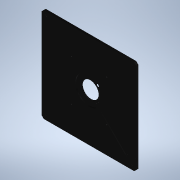
# Autodesk Inventor part: J002949
Saved by Autodesk Inventor 2020.3 (Build 243373000, 373)
## iProperties
RuleStatus: InUse
AfterDocSave0: file://Part Number Cleaner
Created: 2013-12-12
Material: ALUMINUM, 6061-T651
Vendor: HHMI: JFRC - ID&F
Document SubType Name: Modeling
Designer: TABACHNIKT
Density: 2.7 g/cm^3
Mass: 1277.78 g
Surface Area: 1603.58 cm^2
Volume: 473.251 cm^3
Project: P-208804
Description: BASE PLATE
Part Number: J002949
Appearance: Glossy - Black
LAB/DEPT: BRANSON (LAB)
REQUESTING SCIENTIST: ROBIE, ALICE
SURFACE ROUGHNESS: 63 Ra
DESIGN DEPARTMENT: HHMI: JRC - ID&F
SPECIAL FINISH: ANODIZE PER MIL-A-8625F, TYPE II, CLASS 2 (BLACK)
ALTERED ITEM PART NUMBER: N/A
ALTERED ITEM VENDOR: N/A
ALTERED ITEM DESCRIPTION: N/A
PART NUMBER - LEGACY: J002588
Revision Number: A
Autodesk Inventor part; units mm, degrees
ref_plane "YZ Plane" through (0, 0, 0) normal (1, 0, 0) x (0, 1, 0)
ref_plane "XZ Plane" through (0, 0, 0) normal (0, 1, 0) x (-1, 0, 0)
ref_plane "XY Plane" through (0, 0, 0) normal (0, 0, 1) x (1, 0, 0)
sketch "Sketch1" plane through (0, 0, 0) normal (0, 0, 1) x (1, 0, 0)
  line L0 (-152.4, 152.4) -> (152.4, 152.4)
  line L1 (152.4, 152.4) -> (152.4, -152.4)
  line L2 (152.4, -152.4) -> (-152.4, -152.4)
  line L3 (-152.4, -152.4) -> (-152.4, 152.4)
  circle A0 centre (0, 0) radius 26.67
  circle A1 centre (-139.7, 139.7) radius 3.2639
  circle A2 centre (139.7, 139.7) radius 3.2639
  circle A3 centre (139.7, -139.7) radius 3.2639
  circle A4 centre (-139.7, -139.7) radius 3.2639
  point P0 (0, 152.4)
  point P1 (-152.4, 0)
  dimension "d0" = 53.34
  dimension "d1" = 304.8
  dimension "d2" = 304.8
  dimension "d3" = 6.5278
  dimension "d4" = 6.5278
  dimension "d5" = 6.5278
  dimension "d6" = 6.5278
  dimension "d7" = 279.4
  dimension "d8" = 139.7
  dimension "d9" = 279.4
  dimension "d10" = 139.7
  constraints: 8 end point, 5 centre point, 3 horizontal alignment, 3 vertical alignment, 2 midpoint, 2 parallel, 1 coincident, 1 horizontal, 1 perpendicular
  measures "d0" diameter of A0
  measures "d1" distance of L2.end L0.start
  measures "d2" distance of L1.end L2.end
  measures "d3" diameter of A1
  measures "d4" diameter of A2
  measures "d5" diameter of A3
  measures "d6" diameter of A4
  measures "d7" distance of A4.centre A1.centre
  measures "d8" horizontal distance of A4.centre point (0, 0)
  measures "d9" distance of A2.centre A1.centre
  measures "d10" horizontal distance of point (0, 0) A1.centre
extrude "Extrusion1" add sketch "Sketch1" along normal blind 6.35
chamfer "Chamfer1" distance 6.35 angle 45 4 edges at (152.4, 152.4, 3.175) (152.4, -152.4, 3.175) (-152.4, 152.4, 3.175) (-152.4, -152.4, 3.175)
sketch "Sketch10" plane through (0, 0, 6.35) normal (0, 0, 1) x (1, 0, 0)
  line L0 (-213.36, 0) -> (213.36, 0) construction
  line L1 (0, -213.36) -> (0, 213.36) construction
  line L2 (-81.3558, 81.3558) -> (81.3558, -81.3558) construction
  line L3 (15.2664, -26.0427) -> (26.0427, -15.2664) construction
  line L4 (26.0427, -15.2664) -> (33.2269, -22.4506) construction
  line L5 (27.8388, -27.8388) -> (22.4506, -33.2269) construction
  line L6 (22.4506, -33.2269) -> (15.2664, -26.0427) construction
  circle A0 centre (0, 0) radius 26.67 projected
  line L7 (18.8585, -29.6348) -> (29.6348, -18.8585) construction
  line L8 (152.4, 146.05) -> (152.4, -146.05) projected
  line L9 (152.4, -112.6871) -> (120.0658, -112.6871)
  line L10 (116.8908, -115.8621) -> (116.8908, -122.2375)
  line L11 (120.0658, -125.4125) -> (152.4, -125.4125)
  line L12 (152.4, -125.4125) -> (152.4, -112.6871)
  arc A1 (120.0658, -112.6871) -> (116.8908, -115.8621) centre (120.0658, -115.8621) ccw
  arc A2 (116.8908, -122.2375) -> (120.0658, -125.4125) centre (120.0658, -122.2375) ccw
  line L13 (146.05, -152.4) -> (-146.05, -152.4) projected
  line L14 (118.491, -123.8123) -> (150.241, -123.8123) construction
  line L15 (150.241, -123.8123) -> (150.241, -114.2873) construction
  line L16 (150.241, -114.2873) -> (118.491, -114.2873) construction
  line L17 (118.491, -114.2873) -> (118.491, -123.8123) construction
  line L18 (134.366, -114.2873) -> (134.366, -123.8123) construction
  line L19 (118.491, -119.0498) -> (150.241, -119.0498) construction
  arc A3 (33.5957, -29.1055) -> (29.1055, -33.5957) centre (0, 0) ccw
  line L20 (29.1055, -33.5957) -> (116.8908, -121.3809)
  line L21 (33.5957, -29.1055) -> (117.9685, -113.4784)
  line L22 (21.9118, -20.8342) -> (24.0671, -22.9895)
  line L23 (24.0671, -22.9895) -> (22.9895, -24.0671)
  line L24 (22.9895, -24.0671) -> (20.8342, -21.9118)
  line L25 (20.8342, -21.9118) -> (21.9118, -20.8342)
  line L26 (21.373, -21.373) -> (23.5283, -23.5283) construction
  line L27 (20.1158, -22.6302) -> (22.271, -24.7855)
  line L28 (19.0381, -23.7079) -> (20.1158, -22.6302)
  line L29 (21.1934, -25.8631) -> (19.0381, -23.7079)
  line L30 (22.271, -24.7855) -> (21.1934, -25.8631)
  line L31 (22.6302, -20.1158) -> (23.7079, -19.0381)
  line L32 (24.7855, -22.271) -> (22.6302, -20.1158)
  line L33 (23.7079, -19.0381) -> (25.8631, -21.1934)
  line L34 (25.8631, -21.1934) -> (24.7855, -22.271)
  point P0 (22.3249, -22.3249)
  point P1 (20.6546, -27.8388)
  point P2 (27.8388, -20.6546)
  point P3 (121.666, -119.0498)
  point P4 (147.066, -119.0498)
  point P5 (20.5289, -24.121)
  point P6 (24.121, -20.5289)
  point P7 (19.577, -23.1691)
  point P8 (21.7322, -25.3243)
  point P9 (23.1691, -19.577)
  point P10 (25.3243, -21.7322)
  dimension "d84" = 45
  dimension "d85" = 10.16
  dimension "d86" = 15.24
  dimension "d87" = 39.37
  dimension "d90" = 2.3622
  dimension "d91" = 10.16
  dimension "d101" = 3.175
  dimension "d120" = 31.75
  dimension "d121" = 9.525
  dimension "d122" = 25.4
  dimension "d124" = 33.3502
  dimension "d125" = 1.6002
  dimension "d126" = 1.6002
  dimension "d128" = 2.159
  dimension "d156" = 88.9
  dimension "d159" = 6.35
  dimension "d163" = 2.3622
  dimension "d164" = 2.3622
  dimension "d165" = 2.54
  dimension "d166" = 2.54
  dimension "d167" = 3.048
  dimension "d168" = 1.524
  dimension "d172" = 2.54
  dimension "d179" = 2.54
  dimension "d185" = 1.016
  constraints: 62 end point, 11 midpoint, 10 parallel, 9 point on circle, 8 point on line, 6 perpendicular, 4 tangent, 3 centre point, 3 collinear, 2 horizontal, 2 symmetric about line, 1 coincident, 1 equal radius, 23 other
  measures "d84" angle of L0 L2
  measures "d85" distance of L3.end L4.end
  measures "d86" distance of L3.start L3.end
  measures "d87" distance from line of L5 point (0, 0)
  measures "d90" distance from line of point (22.325, -22.325) L3
  measures "d91" distance of point (27.839, -20.655) point (20.655, -27.839)
  measures "d101" radius of A1
  measures "d120" distance of L15.end L16.end
  measures "d121" distance of L16.end L14.start
  measures "d122" distance of point (147.066, -119.05) point (121.666, -119.05)
  measures "d124" distance between parallel lines of L19 L13
  measures "d125" distance between parallel lines of L10 L17
  measures "d126" distance between parallel lines of L16 L9
  measures "d128" distance between parallel lines of L15 L12
  measures "d156" diameter of A3
  measures "d159" distance between parallel lines of L21 L20
  measures "d163" distance from line of L3 point (20.529, -24.121)
  measures "d164" distance from line of L3 point (24.121, -20.529)
  measures "d165" distance of point (22.325, -22.325) point (20.529, -24.121)
  measures "d166" distance of point (24.121, -20.529) point (22.325, -22.325)
  measures "d167" distance of L23.end L24.end
  measures "d168" distance of L24.end L22.start
  measures "d172" distance of L22.start L27.start
  measures "d179" distance of L24.end L31.start
  measures "d185" distance between parallel lines of L7 L30
hole "Hole8" at (22.3249, -22.3249, 6.35) at (20.5289, -24.121, 6.35) at (24.121, -20.5289, 6.35) direction (0, 0, -1) diameter 1.27 end through all
hole "Hole9" at (20.6546, -27.8388, 6.35) at (27.8388, -20.6546, 6.35) at (121.666, -119.0498, 6.35) at (147.066, -119.0498, 6.35) direction (0, 0, -1) diameter 1.7018 end through all
extrude "Extrusion5" cut sketch "Sketch10" against normal blind 3.175 contours A0 | L8 L11 A2 L10 A1 L9 | A1 L10 L20 A3 L21 | L22 L23 L24 L25 | L27 L30 L29 L28 | L31 L33 L34 L32
sketch "Sketch11" plane through (0, 0, 6.35) normal (0, 0, 1) x (1, 0, 0)
  line L0 (-213.36, 0) -> (213.36, 0) construction
  line L1 (0, -213.36) -> (0, 213.36) construction
  line L2 (-84.555, -84.555) -> (84.555, 84.555) construction
  circle A0 centre (22.4506, 22.4506) radius 1.9812 construction
  circle A1 centre (26.0427, 26.0427) radius 0.8509 construction
  circle A2 centre (23.8516, 23.8516) radius 4.9022
  point P0 (0, 0)
  dimension "d130" = 45
  dimension "d135" = 3.9624
  dimension "d136" = 1.7018
  dimension "d142" = 31.75
  dimension "d143" = 5.08
  dimension "d157" = 9.8044
  dimension "d158" = 33.7312
  constraints: 3 centre point, 3 point on line, 2 end point, 1 midpoint
  measures "d130" angle of L2 L0
  measures "d135" diameter of A0
  measures "d136" diameter of A1
  measures "d142" distance of A0.centre point (0, 0)
  measures "d143" distance of A1.centre A0.centre
  measures "d157" diameter of A2
  measures "d158" distance of A2.centre point (0, 0)
extrude "Extrusion6" cut sketch "Sketch11" against normal through all
sketch "Sketch12" plane through (0, 0, 0) normal (0, 0, -1) x (-1, 0, 0)
  line L0 (-57.15, 66.675) -> (57.15, 66.675) construction
  line L1 (57.15, 66.675) -> (57.15, -66.675) construction
  line L2 (57.15, -66.675) -> (-57.15, -66.675) construction
  line L3 (-57.15, -66.675) -> (-57.15, 66.675) construction
  line L4 (-57.15, 66.675) -> (57.15, -66.675) construction
  point P0 (0, 0)
  point P1 (0, 0)
  dimension "d147" = 133.35
  dimension "d148" = 114.3
  constraints: 10 end point, 5 coincident, 2 parallel, 1 horizontal, 1 midpoint, 1 perpendicular
  measures "d147" distance of L0.end L1.end
  measures "d148" distance of L1.end L2.end
hole "Hole10" at (-57.15, 66.675, 0) at (-57.15, -66.675, 0) at (57.15, -66.675, 0) at (57.15, 66.675, 0) direction (0, 0, 1) diameter 3.302 end through all thread size "8-32 UNC" class "2B" standard "ANSI Unified Screw Threads"
chamfer "Chamfer2" distance 1.6002 angle 45 1 edges at (-26.67, 0, 3.175)
extrude "Extrusion7" cut sketch "Sketch10" against normal blind 4.191 contours L22 L23 L24 L25 | L27 L30 L29 L28 | L31 L33 L34 L32
equation "\"d4\" = d3"
equation "\"d5\" = d3"
equation "\"d6\" = d3"
equation "\"d8\" = 0.5 * d7"
equation "\"d10\" = 0.5 * d9"
equation "\"d126\" = d125"
equation "\"d163\" = d90"
equation "\"d164\" = d90"
equation "\"d166\" = d165"
body "Solid1"
